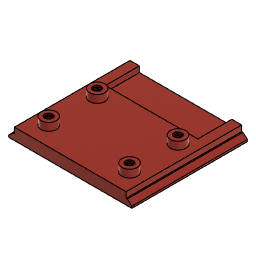
camera-bracket (Autodesk Fusion 360 design; units mm, degrees)
Autodesk Fusion 360 part; units mm, degrees
sketch "Sketch1" plane through (0, 0, 0) normal (0, 0, 1) x (1, 0, 0)
  line L0 (-30.6238, 30.6157) -> (-1.6238, 30.6157)
  line L1 (-1.6238, 30.6157) -> (-1.6238, 0.6157)
  line L2 (-1.6238, 0.6157) -> (-30.6238, 0.6157)
  line L3 (-30.6238, 0.6157) -> (-30.6238, 30.6157)
  line L4 (-28.6238, 25.6157) -> (-28.6238, 5.6157)
  line L5 (-26.6238, 3.6157) -> (-5.6238, 3.6157)
  circle A0 centre (-5.6238, 18.1157) radius 1.05
  line L6 (-27.6738, 18.1157) -> (-4.5738, 18.1157) construction
  circle A1 centre (-5.6238, 5.5357) radius 1.05
  line L7 (-27.6738, 5.5357) -> (-4.5738, 5.5357) construction
  circle A2 centre (-26.6238, 5.5357) radius 1.05
  circle A3 centre (-26.6238, 18.1157) radius 1.05
  line L8 (-26.6238, 4.4857) -> (-26.6238, 19.1657) construction
  line L9 (-5.6238, 5.5357) -> (-5.6238, 18.1157) construction
  circle A4 centre (-26.6238, 5.5357) radius 2
  circle A5 centre (-26.6238, 18.1157) radius 2
  circle A6 centre (-5.6238, 18.1157) radius 2
  circle A7 centre (-5.6238, 5.5357) radius 2
  circle A8 centre (-26.6238, 5.5357) radius 1.05
  circle A9 centre (-26.6238, 18.1157) radius 1.05
  circle A10 centre (-26.6238, 5.5357) radius 1.05
  circle A11 centre (-5.6238, 5.5357) radius 1.05
  circle A12 centre (-5.6238, 18.1157) radius 1.05
  line L10 (-4.1738, 30.6157) -> (-4.1738, 21.7837)
  line L11 (-4.1738, 21.7837) -> (-28.1738, 21.7837)
  line L12 (-28.1738, 21.7837) -> (-28.1738, 30.6157)
  line L13 (-5.1738, 27.6157) -> (-5.1738, 22.1157)
  point P0 (-27.6738, 18.1157)
  point P1 (-27.6738, 5.5357)
  dimension "d1" = 30
  dimension "d2" = 29
  dimension "d3" = 2
  dimension "d4" = 3
  dimension "d5" = 4
  dimension "d6" = 4
  dimension "d7" = 4
  dimension "d8" = 4
  dimension "d9" = 2.1
  dimension "d10" = 2.1
  dimension "d11" = 2.1
  dimension "d12" = 2.1
  dimension "d13" = 8.832
  dimension "d14" = 24
  dimension "d15" = 1
  constraint horizontal L0
  constraint vertical L1
  constraint horizontal L2
  constraint vertical L3
  constraint coincident P0 L6.start
  constraint coincident A0 L6.end
  constraint perpendicular L4 L6
  constraint coincident P1 L7.start
  constraint coincident A1 L7.end
  constraint parallel L6 L7
  constraint coincident A2 L8.start
  constraint coincident A3 L8.end
  constraint perpendicular L6 L8
  constraint coincident A1.centre L9.start
  constraint coincident A0.centre L9.end
  constraint concentric A2 A4
  constraint concentric A3 A5
  constraint concentric A4 A8
  constraint concentric A5 A9
  constraint concentric A8 A10
  constraint concentric A7 A11
  constraint concentric A6 A12
  constraint coincident L0 L10.start
  constraint perpendicular L0 L10
  constraint perpendicular L3 L11
  constraint coincident L0 L12.end
  constraint perpendicular L0 L12
  measures "d1" distance of L0 L2
  measures "d2" distance of L1 L3
  measures "d3" distance of L3 L4
  measures "d4" distance of L2 L5
  measures "d5" diameter of A4
  measures "d6" diameter of A5
  measures "d7" diameter of A6
  measures "d8" diameter of A7
  measures "d9" diameter of A9
  measures "d10" diameter of A10
  measures "d11" diameter of A11
  measures "d12" diameter of A12
  measures "d13" distance of L10.start L10.end
  measures "d14" distance of L10.end L11.end
  measures "d15" distance of L10 L13
extrude "Extrude1" add sketch "Sketch1" along normal blind 3 contours L0 L1 L2 L3 L10 L11 L12 | L0 L10 L11 L12
extrude "Extrude2" add sketch "Sketch1" along normal blind 5 contours A4 | A5 | A6 | A7
extrude "Extrude3" cut sketch "Sketch1" along normal blind 3 contours L0 L10 L11 L12
thread "Thread1" "ISO Metric profile 2.0 M2x0.4 6H" major diameter 2.074 minor diameter 1.623 pitch 0.4 angle 60 modelled right hand crest width 0.05 on face at (-6.6414, 17.8566, 3.3333) crest through (-4.8123, 18.1157, -0.225)
thread "Thread2" "ISO Metric profile 2.0 M2x0.4 6H" major diameter 2.074 minor diameter 1.623 pitch 0.4 angle 60 modelled right hand crest width 0.05 on face at (-4.5751, 5.4834, 3.3333) crest through (-4.8123, 5.5357, -0.225)
thread "Thread3" "ISO Metric profile 2.0 M2x0.4 6H" major diameter 2.074 minor diameter 1.623 pitch 0.4 angle 60 modelled right hand crest width 0.05 on face at (-25.5751, 5.4834, 3.3333) crest through (-25.8123, 5.5357, -0.225)
thread "Thread4" "ISO Metric profile 2.0 M2x0.4 6H" major diameter 2.074 minor diameter 1.623 pitch 0.4 angle 60 modelled right hand crest width 0.05 on face at (-25.5751, 18.0634, 3.3333) crest through (-25.8123, 18.1157, -0.225)
sketch "Sketch2" plane through (-30.6238, 0, 0) normal (-1, 0, 0) x (0, -1, 0)
  line L0 (-30.6157, 0) -> (-0.6157, 0)
  line L1 (-0.6157, 0) -> (-0.6157, 3)
  line L2 (-0.6157, 3) -> (-30.6157, 3)
  line L3 (-30.6157, 3) -> (-30.6157, 0)
  line L4 (-0.6157, 1.5) -> (-30.6157, 1.5)
  constraint midpoint L1 L4.start
  constraint midpoint L3 L4.end
extrude "Extrude4" add sketch "Sketch2" along normal blind 1.5 and the other way blind 30.5 contours L0 L1 L3 L4
chamfer "Chamfer1" distance 1 angle 50 2 edges at (-0.1238, 15.6157, 1.5) (-32.1238, 15.6157, 1.5) measured on face at (-0.1238, 20.6157, 1) measured on face at (-32.1238, 20.6157, 1)
